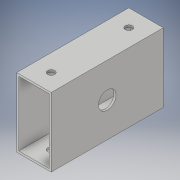
# Autodesk Inventor part: 1x1 Bumper Attachment
Saved by Autodesk Inventor 2018 (Build 220112000, 112)
## iProperties
Created: 2019-01-26
Part Number: 1x1 Bumper Attachment
Material: Generic
Document SubType Name: Modeling
Designer: s-2512711
Density: 1 g/cm^3
Appearance: Default
Author: s-2512711
Autodesk Inventor part; units mm, degrees
ref_plane "YZ Plane" through (0, 0, 0) normal (1, 0, 0) x (0, 1, 0)
ref_plane "XZ Plane" through (0, 0, 0) normal (0, 1, 0) x (-1, 0, 0)
ref_plane "XY Plane" through (0, 0, 0) normal (0, 0, 1) x (1, 0, 0)
sketch "Sketch1" plane through (0, 0, 0) normal (0, 0, 1) x (1, 0, 0)
  line L0 (0, 0) -> (25.4, 0)
  line L1 (25.4, 0) -> (25.4, 50.8)
  line L2 (25.4, 50.8) -> (0, 50.8)
  line L3 (0, 50.8) -> (0, 0)
  line L4 (1.5875, 49.2125) -> (23.8125, 49.2125)
  line L5 (23.8125, 49.2125) -> (23.8125, 1.5875)
  line L6 (23.8125, 1.5875) -> (1.5875, 1.5875)
  line L7 (1.5875, 1.5875) -> (1.5875, 49.2125)
  dimension "d0" = 25.4
  dimension "d1" = 50.8
  dimension "d2" = 1.5875
  constraints: 16 end point, 4 parallel, 2 perpendicular, 1 horizontal, 3 other
  measures "d0" distance of L2.end L1.end
  measures "d1" distance of L1.end L0.end
  measures "d2" distance between parallel lines of L2 L4
extrude "Extrusion1" add sketch "Sketch1" along normal blind 82.55
sketch "Sketch3" plane through (25.4, 0, 0) normal (1, 0, 0) x (0, 0, -1)
  line L0 (0, 50.8) -> (-82.55, 50.8) construction
  line L1 (-41.275, 50.8) -> (-41.275, 25.4) construction
  circle A0 centre (-41.275, 25.4) radius 6.477
  point P0 (0, 0)
  dimension "d10" = 25.4
  dimension "d15" = 12.954
  constraints: 2 coincident, 2 end point, 1 centre point, 1 midpoint, 1 vertical
  measures "d10" distance of L1.start L1.end
  measures "d15" diameter of A0
extrude "Extrusion3" cut sketch "Sketch3" against normal blind 82.55
sketch "Sketch4" plane through (0, 50.8, 0) normal (0, 1, 0) x (1, 0, 0)
  line L0 (1.5875, 0) -> (23.8125, 0) construction
  line L1 (12.7, 0) -> (12.7, -12.7) construction
  line L2 (23.8125, -82.55) -> (1.5875, -82.55) construction
  line L3 (12.7, -82.55) -> (12.7, -69.85) construction
  circle A0 centre (12.7, -69.85) radius 2.5797
  circle A1 centre (12.7, -12.7) radius 2.5797
  point P0 (0, 0)
  dimension "d16" = 12.7
  dimension "d17" = 12.7
  dimension "d18" = 5.1594
  constraints: 4 end point, 2 centre point, 2 coincident, 2 midpoint, 2 vertical
  measures "d16" distance of L1.start L1.end
  measures "d17" distance of L3.start L3.end
  measures "d18" diameter of A0
extrude "Extrusion4" cut sketch "Sketch4" against normal blind 82.55
body "Solid1"
